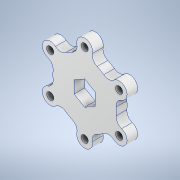
# Autodesk Inventor part: HubPlate
Saved by Autodesk Inventor 2020 (Build 240168000, 168)
## iProperties
Created: 2019-07-10
Part Number: HubPlate
Material: Aluminum 6061
Document SubType Name: Modeling
Designer: Connor
Density: 2.7 g/cm^3
Appearance: Aluminum - Flat
Author: Connor
Autodesk Inventor part; units mm, degrees
ref_plane "YZ Plane" through (0, 0, 0) normal (1, 0, 0) x (0, 1, 0)
ref_plane "XZ Plane" through (0, 0, 0) normal (0, 1, 0) x (-1, 0, 0)
ref_plane "XY Plane" through (0, 0, 0) normal (0, 0, 1) x (1, 0, 0)
sketch "Sketch1" plane through (0, 0, 0) normal (0, 0, 1) x (1, 0, 0)
  line L0 (0, 7.3323) -> (6.35, 3.6662)
  line L1 (6.35, 3.6662) -> (6.35, -3.6662)
  line L2 (6.35, -3.6662) -> (0, -7.3323)
  line L3 (0, -7.3323) -> (-6.35, -3.6662)
  line L4 (-6.35, -3.6662) -> (-6.35, 3.6662)
  line L5 (-6.35, 3.6662) -> (0, 7.3323)
  circle A0 centre (0, 23.8125) radius 2.159
  circle A1 centre (0, 0) radius 19.05
  circle A2 centre (0, 23.8125) radius 4.7625
  circle A3 centre (-20.6222, 11.9063) radius 4.7625
  circle A4 centre (-20.6222, 11.9063) radius 2.159
  circle A5 centre (-20.6222, -11.9062) radius 4.7625
  circle A6 centre (-20.6222, -11.9062) radius 2.159
  circle A7 centre (0, -23.8125) radius 4.7625
  circle A8 centre (0, -23.8125) radius 2.159
  circle A9 centre (20.6222, -11.9063) radius 4.7625
  circle A10 centre (20.6222, -11.9063) radius 2.159
  circle A11 centre (20.6222, 11.9062) radius 4.7625
  circle A12 centre (20.6222, 11.9062) radius 2.159
  arc A13 (-7.466, 17.526) -> (-4.6663, 22.86) centre (-9.3326, 21.9075) ccw
  arc A14 (4.6663, 22.86) -> (7.466, 17.526) centre (9.3326, 21.9075) ccw
  arc A15 (-18.911, 2.2972) -> (-22.1305, 7.3889) centre (-23.6387, 2.8715) ccw
  arc A16 (-17.4642, 15.4711) -> (-11.4449, 15.2288) centre (-14.3062, 19.036) ccw
  arc A17 (-11.4449, -15.2288) -> (-17.4642, -15.4711) centre (-14.3062, -19.036) ccw
  arc A18 (-22.1305, -7.3889) -> (-18.911, -2.2972) centre (-23.6387, -2.8715) ccw
  arc A19 (7.466, -17.526) -> (4.6663, -22.86) centre (9.3326, -21.9075) ccw
  arc A20 (-4.6663, -22.86) -> (-7.466, -17.526) centre (-9.3326, -21.9075) ccw
  arc A21 (18.911, -2.2972) -> (22.1305, -7.3889) centre (23.6387, -2.8715) ccw
  arc A22 (17.4642, -15.4711) -> (11.4449, -15.2288) centre (14.3062, -19.036) ccw
  arc A23 (11.4449, 15.2288) -> (17.4642, 15.4711) centre (14.3062, 19.036) ccw
  arc A24 (22.1305, 7.3889) -> (18.911, 2.2972) centre (23.6387, 2.8715) ccw
  point P0 (0, 19.05)
  point P1 (-3.6714, 18.6929)
  point P2 (-16.4978, 9.525)
  point P3 (-18.0242, 6.1669)
  point P4 (-16.4978, -9.525)
  point P5 (-14.3528, -12.526)
  point P6 (0, -19.05)
  point P7 (3.6714, -18.6929)
  point P8 (16.4978, -9.525)
  point P9 (18.0242, -6.1669)
  point P10 (16.4978, 9.525)
  point P11 (14.3528, 12.526)
  point P12 (22.1305, 7.3889)
  point P13 (11.4449, -15.2288)
  point P14 (17.4642, -15.4711)
  point P15 (22.1305, -7.3889)
  point P16 (-7.466, -17.526)
  point P17 (-4.6663, -22.86)
  point P18 (4.6663, -22.86)
  point P19 (-18.911, -2.2972)
  point P20 (-22.1305, -7.3889)
  point P21 (-17.4642, -15.4711)
  point P22 (-11.4449, -15.2288)
  point P23 (-11.4449, 15.2288)
  point P24 (-22.1305, 7.3889)
  dimension "d0" = 12.7
  dimension "d1" = 4.318
  dimension "d2" = 38.1
  dimension "d3" = 9.525
  dimension "d6" = 360
  dimension "d11" = 23.8125
  dimension "d14" = 360
  constraints: 28 point on circle, 25 centre point, 12 end point, 8 coincident, 4 tangent, 2 equal radius, 2 vertical alignment, 87 other
  measures "d0" distance between parallel lines of L1 L4
  measures "d1" diameter of A0
  measures "d2" diameter of A1
  measures "d3" diameter of A2
  measures "d11" distance of point (0, 0) A0.centre
extrude "Extrusion1" add sketch "Sketch1" along normal blind 6.35
body "Solid1"
